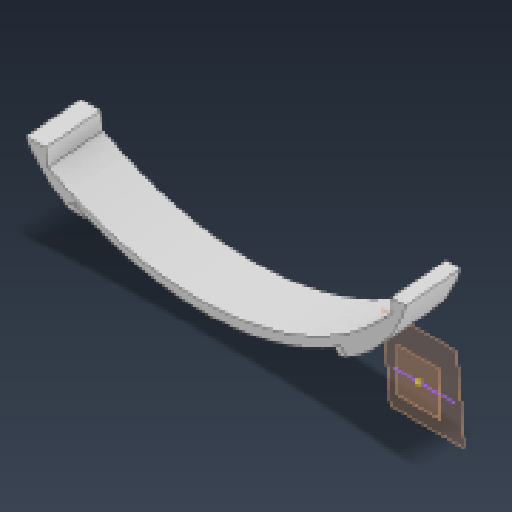
# Autodesk Inventor part: thigh_strap_02
Saved by Autodesk Inventor 2025.2 (Build 292293000, 293)
## iProperties
Created: 2025-03-07
Part Number: thigh_strap_02
Material: Generic
Document SubType Name: Modeling
Designer: email
Density: 1 g/cm^3
Appearance: Default
Author: email
Autodesk Inventor part; units mm, degrees
ref_plane "YZ Plane" through (0, 0, 0) normal (1, 0, 0) x (0, 1, 0)
ref_plane "XZ Plane" through (0, 0, 0) normal (0, 1, 0) x (-1, 0, 0)
ref_plane "Work Plane1" through (0, 0, -50.8) normal (0, 0, 1) x (1, 0, 0)
sketch "Sketch1" plane through (0, 0, -50.8) normal (0, 0, 1) x (1, 0, 0)
  line L0 (-11.933319, 0) -> (16.362179, 0)
  point P0 (0, 0)
  constraints: 2 end point, 1 horizontal
ref_plane "Work Plane2" through (-11.933319, 0, -50.8) normal (0, -0.0871557, 0.9961947) x (1, 0, 0)
sketch "Sketch2" plane through (-11.933319, 0, -50.8) normal (0, -0.0871557, 0.9961947) x (1, 0, 0)
  line L0 (20.901803, 66.92299) -> (20.901803, 43.564038)
  line L1 (18.251803, 42.008516) -> (18.251803, 68.335864)
  line L2 (18.251803, 42.008516) -> (20.901803, 42.008516)
  line L3 (-146.748197, 17.044024) -> (-146.748197, 40.704766)
  line L4 (-149.398197, 17.044024) -> (-149.398197, 40.704766)
  line L5 (-149.398197, 42.001169) -> (-149.398197, 42.510921)
  line L6 (-146.748197, 17.044024) -> (-149.398197, 17.044024)
  arc A0 (-146.748197, 17.044024) -> (18.251803, 42.008516) centre (-77.743959, 118.72499) ccw
  arc A1 (-149.398197, 17.044024) -> (20.901803, 42.008516) centre (-75.863874, 108.764811) ccw
  line L7 (-121.884258, 0.588457) -> (-124.244108, -1.791919)
  arc A2 (-154.040418, 23.398782) -> (-124.244108, -1.791919) centre (-114.93586, 39.435485) ccw
  line L8 (-154.040418, 23.398782) -> (-144.892983, 23.398782)
  line L9 (-144.892983, 23.398782) -> (-144.394088, 15.485637)
  line L10 (-21.699981, 4.427512) -> (-19.714804, 2.459452)
  arc A3 (-19.714804, 2.459452) -> (22.454201, 45.29191) centre (-43.243229, 67.797577) ccw
  line L11 (22.454201, 45.29191) -> (15.711222, 45.29191)
  line L12 (15.711222, 45.29191) -> (15.711222, 38.933181)
  point P0 (11.933319, 4.427512)
extrude "Extrusion1" add sketch "Sketch2" along normal mid plane 25.4
fillet "Fillet1" radius 12.7 4 edges at (-32.6407, 2.3235, -37.8482) (-32.6407, 4.5373, -63.1516) (-134.9975, -1.7063, -38.2008) (-134.9975, 0.5074, -63.5041)
body "Solid1"
